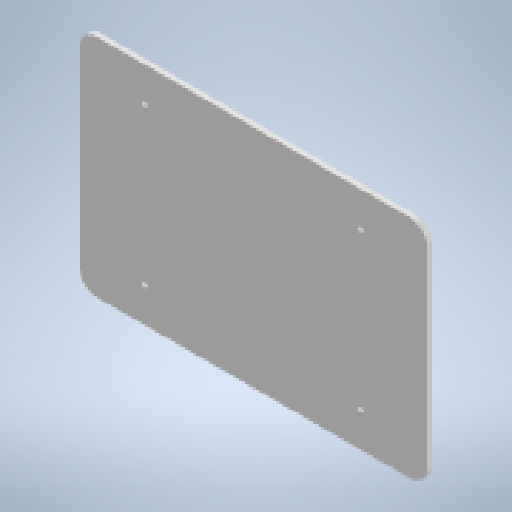
# Autodesk Inventor part: Bottom layer2
Saved by Autodesk Inventor 2023 (Build 270158000, 158)
## iProperties
Created: 2024-10-04
Part Number: Bottom layer2
Material: Generic
Document SubType Name: Modeling
Designer: bw1293
Density: 1 g/cm^3
Appearance: Default
Author: bw1293
Autodesk Inventor part; units mm, degrees
ref_plane "YZ Plane" through (0, 0, 0) normal (1, 0, 0) x (0, 1, 0)
ref_plane "XZ Plane" through (0, 0, 0) normal (0, 1, 0) x (-1, 0, 0)
ref_plane "XY Plane" through (0, 0, 0) normal (0, 0, 1) x (1, 0, 0)
ref_plane "Work Plane1" through (0, 0, 3) normal (0, 0, 1) x (1, 0, 0)
sketch "Sketch2" plane through (0, 0, 3) normal (0, 0, 1) x (1, 0, 0)
  line L0 (0, 33) -> (12.6, 33)
  line L1 (0, 33) -> (-12.6, 33)
  circle A0 centre (12.6, 33) radius 1.5
  circle A1 centre (-12.6, 33) radius 1.5
  circle A2 centre (12.6, -33) radius 1.5
  circle A3 centre (-12.6, -33) radius 1.5
  line L2 (90, 0) -> (47.5, 0)
  line L3 (47.5, 0) -> (47.5, -30)
  circle A4 centre (47.5, -30) radius 1.5
  line L4 (47.5, -30) -> (47.5, -10.075)
  line L5 (47.5, -10.075) -> (44.35, -10.075)
  line L6 (44.35, -10.075) -> (44.35, -3.875)
  line L7 (44.35, -3.875) -> (47.5, -3.875)
  line L8 (47.5, -3.875) -> (47.5, -10.075)
  line L9 (47.5, -10.075) -> (50.65, -10.075)
  line L10 (50.65, -10.075) -> (50.65, -3.875)
  line L11 (50.65, -3.875) -> (47.5, -3.875)
  line L12 (47.5, -3.875) -> (47.5, -10.075)
  line L13 (18, -27.5) -> (-18, -27.5)
  line L14 (-20, -25.5) -> (-20, 25.5)
  line L15 (-18, 27.5) -> (18, 27.5)
  line L16 (20, 25.5) -> (20, -25.5)
  line L17 (20, -27.5) -> (-20, 27.5) construction
  line L18 (-20, -27.5) -> (20, 27.5) construction
  line L19 (12.6, -61) -> (0, -61)
  line L20 (0, -61) -> (-25, -61)
  line L21 (-27, -59) -> (-27, -49)
  line L22 (-25, -47) -> (0, -47)
  line L23 (0, -47) -> (0, -61)
  line L24 (0, -47) -> (25, -47)
  line L25 (27, -49) -> (27, -59)
  line L26 (25, -61) -> (0, -61)
  line L27 (0, -61) -> (0, -47)
  line L28 (0, 61) -> (-25, 61)
  line L29 (-27, 59) -> (-27, 49)
  line L30 (-25, 47) -> (0, 47)
  line L31 (0, 47) -> (25, 47)
  line L32 (27, 49) -> (27, 59)
  line L33 (25, 61) -> (0, 61)
  arc A5 (-27, -59) -> (-25, -61) centre (-25, -59) ccw
  arc A6 (-25, -47) -> (-27, -49) centre (-25, -49) ccw
  arc A7 (25, -61) -> (27, -59) centre (25, -59) ccw
  arc A8 (27, -49) -> (25, -47) centre (25, -49) ccw
  arc A9 (25, 47) -> (27, 49) centre (25, 49) ccw
  arc A10 (27, 59) -> (25, 61) centre (25, 59) ccw
  arc A11 (-27, 49) -> (-25, 47) centre (-25, 49) ccw
  arc A12 (-25, 61) -> (-27, 59) centre (-25, 59) ccw
  arc A13 (20, 25.5) -> (18, 27.5) centre (18, 25.5) ccw
  arc A14 (18, -27.5) -> (20, -25.5) centre (18, -25.5) ccw
  arc A15 (-20, -25.5) -> (-18, -27.5) centre (-18, -25.5) ccw
  arc A16 (-18, 27.5) -> (-20, 25.5) centre (-18, 25.5) ccw
  circle A17 centre (47.5, 5.6103) radius 1.5
  line L34 (50.65, 25.5353) -> (50.65, 31.7353)
  line L35 (47.5, 25.5353) -> (50.65, 25.5353)
  line L36 (47.5, 25.5353) -> (44.35, 25.5353)
  line L37 (44.35, 25.5353) -> (44.35, 31.7353)
  line L38 (44.35, 31.7353) -> (47.5, 31.7353)
  line L39 (50.65, 31.7353) -> (47.5, 31.7353)
  line L40 (60, 0) -> (60, -7.7)
  line L41 (60, 0) -> (60, 7.7)
  circle A18 centre (60, -7.7) radius 1.27
  circle A19 centre (60, 7.7) radius 1.27
  line L42 (-60, 0) -> (-60, 7.7)
  line L43 (-60, 0) -> (-60, -7.7)
  circle A20 centre (-60, 7.7) radius 1.27
  circle A21 centre (-60, -7.7) radius 1.27
  circle A22 centre (-60, 0) radius 12.5
  circle A23 centre (60, 0) radius 12.5
  line L44 (47.5, 5.6103) -> (47.5, 31.7353)
  circle A24 centre (61.75, -45) radius 1.5 projected
  circle A25 centre (61.75, 45) radius 1.5 projected
  circle A26 centre (-62.75, 45) radius 1.5 projected
  circle A27 centre (-62.75, -45) radius 1.5 projected
  line L45 (72.5, 0) -> (77.5, 0)
  line L46 (77.5, 0) -> (77.5, -55)
  line L47 (77.5, 0) -> (77.5, 55)
  line L48 (-72.5, 0) -> (-77.5, 0)
  line L49 (-77.5, 0) -> (-77.5, -55)
  line L50 (-77.5, 0) -> (-77.5, 55)
  line L51 (-67.5, -65) -> (67.5, -65)
  line L52 (67.5, 65) -> (-67.5, 65)
  arc A28 (-77.5, -55) -> (-67.5, -65) centre (-67.5, -55) ccw
  arc A29 (-67.5, 65) -> (-77.5, 55) centre (-67.5, 55) ccw
  arc A30 (77.5, 55) -> (67.5, 65) centre (67.5, 55) ccw
  arc A31 (67.5, -65) -> (77.5, -55) centre (67.5, -55) ccw
  line L53 (-12.6, -33) -> (12.6, -33)
  point P0 (0, 0)
  point P1 (-27, -47)
  point P2 (-27, -61)
  point P3 (27, -61)
  point P4 (27, -47)
  point P5 (-27, 47)
  point P6 (-27, 61)
  point P7 (27, 61)
  point P8 (27, 47)
  point P9 (48.1158, -3.875)
  point P10 (12.5, 47)
  point P11 (12.5, 61)
  point P12 (12.5, -61)
  dimension "d36" = 25
  dimension "d37" = 25
  dimension "d5" = 3
  dimension "d6" = 3
  dimension "d7" = 25.2
  dimension "d10" = 30
  dimension "d11" = 3
  dimension "d12" = 19.925
  dimension "d13" = 3.15
  dimension "d14" = 6.2
  dimension "d15" = 3.15
  dimension "d16" = 6.2
  dimension "d17" = 40
  dimension "d18" = 55
  dimension "d21" = 27
  dimension "d22" = 27
  dimension "d24" = 2
  dimension "d27" = 60
  dimension "d28" = 7.7
  dimension "d29" = 7.7
  dimension "d30" = 2.54
  dimension "d31" = 2.54
  dimension "d32" = 7.7
  dimension "d33" = 7.7
  dimension "d34" = 2.54
  dimension "d35" = 2.54
  dimension "d39" = 5
  dimension "d40" = 5
  dimension "d41" = 10
  dimension "d43" = 30
  dimension "d44" = 30
  dimension "d47" = 32
  dimension "d48" = 14
  dimension "d50" = 4
  dimension "d58" = 32
  constraints: 108 end point, 32 point on circle, 32 tangent, 29 point on line, 26 centre point, 14 equal radius, 10 parallel, 9 coincident, 9 horizontal, 9 perpendicular, 5 midpoint, 5 vertical, 1 horizontal alignment, 5 other
  measures "d5" diameter of A0
  measures "d6" diameter of A1
  measures "d7" distance of L0.end L1.end
  measures "d10" distance of L2.end L3.end
  measures "d11" diameter of A4
  measures "d12" distance of L4.start L4.end
  measures "d13" distance of L6.end L7.end
  measures "d14" distance of L5.end L6.end
  measures "d15" distance of L11.end L10.end
  measures "d16" distance of L10.end L9.end
  measures "d17" distance of L17.end L18.end
  measures "d18" distance of L18.start L17.end
  measures "d21" distance of point (-27, -47) L22.end
  measures "d22" distance of point (27, -61) L26.end
  measures "d24" radius of A5
  measures "d27" distance of point (0, 0) L42.start
  measures "d28" distance of L40.start L40.end
  measures "d29" distance of L40.start L41.end
  measures "d30" diameter of A18
  measures "d31" diameter of A19
  measures "d32" distance of L42.start L42.end
  measures "d33" distance of L42.start L43.end
  measures "d34" diameter of A20
  measures "d35" diameter of A21
  measures "d39" distance of L45.start L45.end
  measures "d40" distance of L48.start L48.end
  measures "d41" radius of A28
  measures "d43" distance between parallel lines of L46 L4
  measures "d44" distance between parallel lines of L47 L44
  measures "d47" distance between parallel lines of L52 L1
  measures "d48" distance of point (12.5, 47) point (12.5, 61)
  measures "d50" distance between parallel lines of L52 L33
  measures "d58" distance between parallel lines of L51 L53
extrude "Extrusion7" add sketch "Sketch2" along normal blind 3 contours A23 L10 L11 L2 | L2 A23 A17 | A23 L11 L3 | A22 | L46 A31 L51 A28 L49 L50 A29 L52 A30 L47
body "Solid7"
